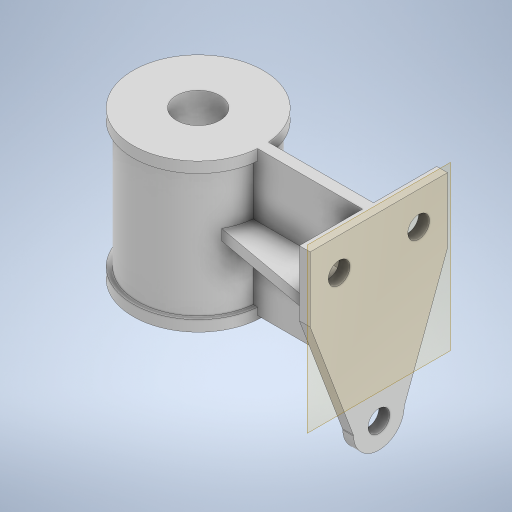
# Autodesk Inventor part: 6 - Part 2
Saved by Autodesk Inventor 2024 (Build 280153000, 153)
## iProperties
Created: 2024-04-21
Part Number: 6 - Part 2
Material: Generic
Document SubType Name: Modeling
Designer: Ricsi
Density: 1 g/cm^3
Appearance: Default
Author: Ricsi
Autodesk Inventor part; units mm, degrees
ref_plane "XZ Plane" through (0, 0, 0) normal (0, 1, 0) x (-1, 0, 0)
ref_plane "XY Plane" through (0, 0, 0) normal (0, 0, 1) x (1, 0, 0)
sketch "Sketch1" plane through (0, 0, 0) normal (0, 1, 0) x (-1, 0, 0)
  circle A0 centre (0, 0) radius 36
  dimension "d0" = 72
  constraints: 1 centre point, 1 coincident
  measures "d0" diameter of A0
extrude "Extrusion1" add sketch "Sketch1" along normal blind 6
sketch "Sketch2" plane through (0, 6, 0) normal (0, 1, 0) x (1, 0, 0)
  circle A0 centre (0, 0) radius 33.5
  dimension "d3" = 67
  constraints: 1 centre point, 1 coincident
  measures "d3" diameter of A0
extrude "Extrusion2" add sketch "Sketch2" along normal blind 70
sketch "Sketch3" plane through (0, 76, 0) normal (0, 1, 0) x (1, 0, 0)
  circle A0 centre (0, 0) radius 36
  dimension "d6" = 72
  constraints: 1 centre point, 1 coincident
  measures "d6" diameter of A0
extrude "Extrusion3" add sketch "Sketch3" along normal blind 6
sketch "Sketch4" plane through (0, 82, 0) normal (0, 1, 0) x (1, 0, 0)
  circle A0 centre (0, 0) radius 12
  dimension "d9" = 24
  constraints: 1 centre point, 1 coincident
  measures "d9" diameter of A0
extrude "Extrusion4" cut sketch "Sketch4" against normal blind 82
ref_plane "Work Plane1" through (100, 0, 0) normal (1, 0, 0) x (0, 1, 0)
sketch "Sketch5" plane through (100, 0, 0) normal (1, 0, 0) x (0, 1, 0)
  line L0 (82, 0) -> (82, 38)
  line L1 (82, 38) -> (46, 38)
  line L2 (82, 38) -> (82, -38)
  line L3 (46, -38) -> (82, -38)
  circle A0 centre (-18, 0) radius 6
  arc A1 (-18.3276, 13.9962) -> (-18.3276, -13.9962) centre (-18, 0) ccw
  line L4 (-17.6721, 14.123) -> (46, 38)
  line L5 (-17.6721, -14.123) -> (46, -38)
  arc A2 (-18.3276, 13.9962) -> (-17.6721, 14.123) centre (-18.3743, 15.9956) ccw
  arc A3 (-17.6721, -14.123) -> (-18.3276, -13.9962) centre (-18.3743, -15.9956) ccw
  line L6 (82, 38) -> (82, 22)
  circle A4 centre (64, 22) radius 6
  circle A5 centre (64, -22) radius 6
  point P0 (0, 0)
  point P1 (-18, 14)
  point P2 (-18, -14)
  dimension "d16" = 76
  dimension "d17" = 36
  dimension "d18" = 76
  dimension "d21" = 12
  dimension "d22" = 28
  dimension "d23" = 2
  dimension "d24" = 2
  dimension "d27" = 12
  dimension "d28" = 12
  dimension "d29" = 18
  dimension "d30" = 16
  constraints: 14 end point, 8 point on circle, 6 centre point, 4 point on line, 4 tangent, 2 horizontal, 1 coincident
  measures "d16" distance of L0.end L2.end
  measures "d17" distance of L0.end L1.end
  measures "d18" distance of L1.end L3.start
  measures "d21" diameter of A0
  measures "d22" diameter of A1
  measures "d23" radius of A2
  measures "d24" radius of A3
  measures "d27" diameter of A4
  measures "d28" diameter of A5
  measures "d29" distance from line of L2 A5.centre
  measures "d30" distance from line of L3 A5.centre
extrude "Extrusion5" add sketch "Sketch5" against normal blind 6
sketch "Sketch6" plane through (94, 0, 0) normal (-1, 0, 0) x (0, 0, 1)
  line L0 (-38, 82) -> (0, 82)
  line L1 (0, 82) -> (3, 82)
  line L2 (0, 82) -> (-3, 82)
  line L3 (-3, 82) -> (-3, 47)
  line L4 (3, 47) -> (3, 82)
  line L5 (-3, 82) -> (3, 82)
  line L6 (38, 82) -> (-38, 82) projected
  line L7 (-38, 82) -> (0, 82)
  arc A0 (-13.9962, -18.3276) -> (13.9962, -18.3276) centre (0, -18) ccw projected
  line L8 (-3, 47) -> (-3, 2)
  line L9 (3, 47) -> (3, 2)
  line L10 (-3, 2) -> (3, 2)
  point P0 (0, 0)
  dimension "d36" = 35
  dimension "d37" = 6
  dimension "d38" = 38
  dimension "d42" = 45
  constraints: 20 end point, 3 vertical, 2 collinear, 1 horizontal
  measures "d36" distance of L2.end L3.end
  measures "d37" distance of L3.end L4.start
  measures "d38" distance of L0.start L0.end
  measures "d42" distance of L4.start L9.end
extrude "Extrusion6" add sketch "Sketch6" along normal blind 61.25
sketch "Sketch7" plane through (94, 2, -3) normal (0, 0, -1) x (-1, 0, 0)
  line L0 (65, 39) -> (65, 45)
  line L1 (94, 39) -> (94, 45)
  line L2 (0, 80) -> (0, 45)
  line L3 (0, 45) -> (0, 39)
  line L4 (0, 45) -> (94, 45)
  line L5 (0, 39) -> (94, 39)
  line L6 (0, 80) -> (0, 0) projected
  line L7 (94, 39) -> (94, 45)
  point P0 (94, -2)
  dimension "d54" = 6
  dimension "d55" = 94
  dimension "d56" = 94
  constraints: 14 end point, 2 vertical, 1 horizontal, 1 perpendicular
  measures "d54" distance of L2.end L3.end
  measures "d55" distance of L2.end L1.end
  measures "d56" distance of L3.end L1.start
extrude "Extrusion7" add sketch "Sketch7" along normal blind 25 contours L5 L3 L4 L0
sketch "Sketch8" plane through (94, 2, 3) normal (0, 0, 1) x (1, 0, 0)
  line L0 (0, 80) -> (0, 45)
  line L1 (0, 45) -> (0, 39)
  line L2 (0, 45) -> (-94, 45)
  line L3 (0, 39) -> (-94, 39)
  line L4 (0, 39) -> (94, 39) construction
  line L5 (-94, 45) -> (-94, 39)
  line L6 (-58.1252, 4) -> (-130, 4) projected
  point P0 (-94, -2)
  dimension "d60" = 6
  dimension "d61" = 94
  dimension "d62" = 94
  dimension "d63" = 180
  dimension "d64" = 6
  constraints: 12 end point, 3 horizontal, 1 collinear, 1 perpendicular
  measures "d60" distance of L0.end L1.end
  measures "d61" distance of L0.end L2.end
  measures "d62" distance of L1.end L3.end
  measures "d63" angle of L3 L4
  measures "d64" distance of L2.end L3.end
extrude "Extrusion8" add sketch "Sketch8" along normal blind 25
sketch "Sketch9" plane through (33.3654, 47, 3) normal (0, 1, 0) x (1, 0, 0)
  line L0 (0, 0) -> (60.6346, 0) projected
  line L1 (60.6346, -25) -> (-14.9738, -25) projected
  arc A0 (0, 6) -> (0, 0) centre (-33.3654, 3) ccw projected
  line L2 (0, -14) -> (60.6346, -25)
  line L3 (60.6346, -25) -> (-14.9738, -25)
  arc A1 (-14.9738, -25) -> (-4.0764, -13.2605) centre (-33.3654, 3) ccw
  line L4 (60.6346, -25) -> (-4.0764, -13.2605)
  point P0 (-4.0764, -13.2605)
  dimension "d67" = 14
  constraints: 7 end point, 2 point on circle, 2 point on line, 1 centre point, 1 coincident, 1 concentric
  measures "d67" distance of L0.start L2.start
extrude "Extrusion9" cut sketch "Sketch9" against normal blind 14
sketch "Sketch10" plane through (33.3654, 47, -3) normal (0, 1, 0) x (1, 0, 0)
  line L0 (-4.3654, 25) -> (-4.3654, 13.7705)
  line L1 (-4.3654, 13.7705) -> (60.6346, 25)
  line L2 (60.6346, 25) -> (-4.3654, 25) projected
  line L3 (60.6346, 25) -> (-4.3654, 25)
  point P0 (-33.3654, -3)
  constraints: 6 end point, 1 collinear
extrude "Extrusion10" cut sketch "Sketch10" against normal blind 14
equation "\"d68\" = d67"
equation "\"d70\" = d67"
body "Solid1"
